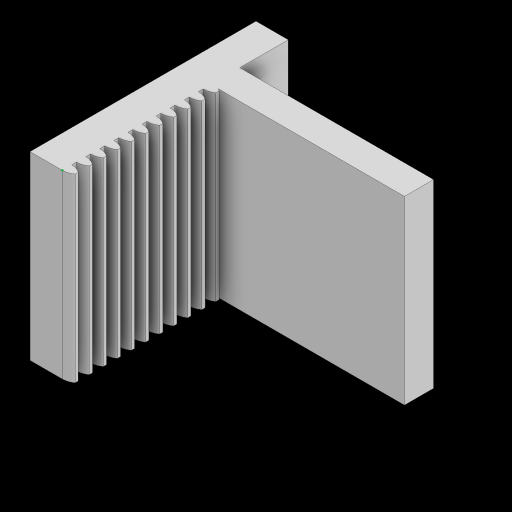
# Autodesk Inventor part: stopper
Saved by Autodesk Inventor 2023 (Build 270158000, 158)
## iProperties
Created: 2024-07-10
Part Number: stopper
Material: 일반
Document SubType Name: Modeling
Designer: OMS55
Density: 1 g/cm^3
Appearance: 기본값
Author: OMS55
Autodesk Inventor part; units mm, degrees
ref_plane "YZ Plane" through (0, 0, 0) normal (1, 0, 0) x (0, 1, 0)
ref_plane "XZ Plane" through (0, 0, 0) normal (0, 1, 0) x (-1, 0, 0)
ref_plane "XY Plane" through (0, 0, 0) normal (0, 0, 1) x (1, 0, 0)
sketch "스케치1" plane through (0, 0, 0) normal (1, 0, 0) x (0, 1, 0)
  line L0 (0, 0) -> (0, -35)
  line L1 (0, -35) -> (-28, -35)
  line L2 (-28, -35) -> (-28, 0)
  line L3 (-28, 0) -> (0, 0)
  line L4 (0, -23) -> (-28, -23)
  line L5 (-28, -23) -> (-28, -27.5)
  line L6 (-28, -27.5) -> (0, -27.5)
  line L7 (0, -27.5) -> (0, -23)
  point P0 (0, -27.5)
  dimension "d0" = 35
  dimension "d1" = 28
  dimension "d2" = 7.5
  dimension "d3" = 4.5
  constraints: 16 end point, 4 parallel, 3 perpendicular, 2 point on line, 1 vertical
  measures "d0" distance of L0.start L0.end
  measures "d1" distance of L2.end L0.start
  measures "d2" distance between parallel lines of L1 L6
  measures "d3" distance between parallel lines of L6 L4
extrude "돌출1" add sketch "스케치1" along normal blind 5 contours L0 L1 L2 L6
extrude "돌출2" add sketch "스케치1" along normal blind 35 contours L0 L6 L2 L4
extrude "돌출3" add sketch "스케치1" along normal blind 5 contours L0 L4 L2 L3
sketch "스케치2" plane through (5, 0, 0) normal (1, 0, 0) x (0, 0, -1)
  point P0 (0, 0)
sketch "스케치3" plane through (0, -28, -35) normal (0, -1, 0) x (1, 0, 0)
  line L0 (0, 35) -> (5, 35) projected
  arc A0 (6.5, 34.523) -> (5, 35) centre (5, 32.403) ccw
  arc A1 (5, 33.546) -> (6.5, 34.023) centre (5, 36.143) ccw
  line L1 (5, 35) -> (9.1174, 35) construction
  line L2 (5, 33.546) -> (9.1174, 33.546) construction
  line L3 (5, 35) -> (5, 12) construction
  line L4 (6.5, 34.523) -> (6.5, 34.023)
  line L5 (5, 35) -> (5, 33.546)
  arc A2 (6.5, 32.342) -> (5, 32.819) centre (5, 30.222) ccw
  arc A3 (5, 31.365) -> (6.5, 31.842) centre (5, 33.962) ccw
  line L6 (5, 32.819) -> (9.1174, 32.819) construction
  line L7 (5, 31.365) -> (9.1174, 31.365) construction
  line L8 (6.5, 32.342) -> (6.5, 31.842)
  line L9 (5, 32.819) -> (5, 31.365)
  arc A4 (6.5, 30.161) -> (5, 30.638) centre (5, 28.041) ccw
  arc A5 (5, 29.184) -> (6.5, 29.661) centre (5, 31.781) ccw
  line L10 (5, 30.638) -> (9.1174, 30.638) construction
  line L11 (5, 29.184) -> (9.1174, 29.184) construction
  line L12 (6.5, 30.161) -> (6.5, 29.661)
  line L13 (5, 30.638) -> (5, 29.184)
  arc A6 (6.5, 27.98) -> (5, 28.457) centre (5, 25.86) ccw
  arc A7 (5, 27.003) -> (6.5, 27.48) centre (5, 29.6) ccw
  line L14 (5, 28.457) -> (9.1174, 28.457) construction
  line L15 (5, 27.003) -> (9.1174, 27.003) construction
  line L16 (6.5, 27.98) -> (6.5, 27.48)
  line L17 (5, 28.457) -> (5, 27.003)
  arc A8 (6.5, 25.799) -> (5, 26.276) centre (5, 23.679) ccw
  arc A9 (5, 24.822) -> (6.5, 25.299) centre (5, 27.419) ccw
  line L18 (5, 26.276) -> (9.1174, 26.276) construction
  line L19 (5, 24.822) -> (9.1174, 24.822) construction
  line L20 (6.5, 25.799) -> (6.5, 25.299)
  line L21 (5, 26.276) -> (5, 24.822)
  arc A10 (6.5, 23.618) -> (5, 24.095) centre (5, 21.498) ccw
  arc A11 (5, 22.641) -> (6.5, 23.118) centre (5, 25.238) ccw
  line L22 (5, 24.095) -> (9.1174, 24.095) construction
  line L23 (5, 22.641) -> (9.1174, 22.641) construction
  line L24 (6.5, 23.618) -> (6.5, 23.118)
  line L25 (5, 24.095) -> (5, 22.641)
  arc A12 (6.5, 21.437) -> (5, 21.914) centre (5, 19.317) ccw
  arc A13 (5, 20.46) -> (6.5, 20.937) centre (5, 23.057) ccw
  line L26 (5, 21.914) -> (9.1174, 21.914) construction
  line L27 (5, 20.46) -> (9.1174, 20.46) construction
  line L28 (6.5, 21.437) -> (6.5, 20.937)
  line L29 (5, 21.914) -> (5, 20.46)
  arc A14 (6.5, 19.256) -> (5, 19.733) centre (5, 17.136) ccw
  arc A15 (5, 18.279) -> (6.5, 18.756) centre (5, 20.876) ccw
  line L30 (5, 19.733) -> (9.1174, 19.733) construction
  line L31 (5, 18.279) -> (9.1174, 18.279) construction
  line L32 (6.5, 19.256) -> (6.5, 18.756)
  line L33 (5, 19.733) -> (5, 18.279)
  arc A16 (6.5, 17.075) -> (5, 17.552) centre (5, 14.955) ccw
  arc A17 (5, 16.098) -> (6.5, 16.575) centre (5, 18.695) ccw
  line L34 (5, 17.552) -> (9.1174, 17.552) construction
  line L35 (5, 16.098) -> (9.1174, 16.098) construction
  line L36 (6.5, 17.075) -> (6.5, 16.575)
  line L37 (5, 17.552) -> (5, 16.098)
  arc A18 (6.5, 14.894) -> (5, 15.371) centre (5, 12.774) ccw
  arc A19 (5, 13.917) -> (6.5, 14.394) centre (5, 16.514) ccw
  line L38 (5, 15.371) -> (9.1174, 15.371) construction
  line L39 (5, 13.917) -> (9.1174, 13.917) construction
  line L40 (6.5, 14.894) -> (6.5, 14.394)
  line L41 (5, 15.371) -> (5, 13.917)
  arc A20 (6.5, 12.713) -> (5, 13.19) centre (5, 10.593) ccw
  arc A21 (5, 11.736) -> (6.5, 12.213) centre (5, 14.333) ccw
  line L42 (5, 13.19) -> (9.1174, 13.19) construction
  line L43 (5, 11.736) -> (9.1174, 11.736) construction
  line L44 (6.5, 12.713) -> (6.5, 12.213)
  line L45 (5, 13.19) -> (5, 11.736)
  point P0 (6.5, 34.273)
  point P1 (5, 34.273)
  point P2 (6.5, 32.092)
  point P3 (5, 32.092)
  point P4 (6.5, 29.911)
  point P5 (5, 29.911)
  point P6 (6.5, 27.73)
  point P7 (5, 27.73)
  point P8 (6.5, 25.549)
  point P9 (5, 25.549)
  point P10 (6.5, 23.368)
  point P11 (5, 23.368)
  point P12 (6.5, 21.187)
  point P13 (5, 21.187)
  point P14 (6.5, 19.006)
  point P15 (5, 19.006)
  point P16 (6.5, 16.825)
  point P17 (5, 16.825)
  point P18 (6.5, 14.644)
  point P19 (5, 14.644)
  point P20 (6.5, 12.463)
  point P21 (5, 12.463)
  dimension "d10" = 1.454
  dimension "d11" = 0.5
  dimension "d12" = 1.5
  dimension "d15" = 2.181
  constraints: 88 end point, 44 point on circle, 22 centre point, 3 vertical, 2 horizontal, 2 midpoint, 2 tangent, 1 horizontal alignment, 1 point on line, 1 vertical alignment, 160 other
  measures "d10" distance of L2.start L0.end
  measures "d11" distance of L4.start L4.end
  measures "d12" distance between parallel lines of L3 L4
  measures "d15" distance of L4.start L8.start
extrude "돌출4" add sketch "스케치3" against normal up to surface (28 mm away)
